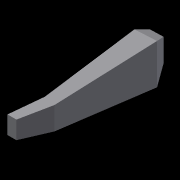
# Autodesk Inventor part: DistalPhalangeIndexMiddle
Saved by Autodesk Inventor 2015 (Build 190159000, 159)
## iProperties
RuleStatus: InUse
Created: 2014-10-29
Part Number: DistalPhalangeIndexMiddle
Material: Generic
Document SubType Name: Modeling
Designer: Val
Density: 1 g/cm^3
Appearance: Default
Mass: 0.761858 g
Surface Area: 6.75236 cm^2
Volume: 0.761858 cm^3
BeforeDocSave0: UpdateBoundingBox
CX: 5.00 mm
CY: 32.00 mm
CZ: 9.00 mm
Author: Val
Autodesk Inventor part; units mm, degrees
ref_plane "YZ Plane" through (0, 0, 0) normal (1, 0, 0) x (0, 1, 0)
ref_plane "XZ Plane" through (0, 0, 0) normal (0, 1, 0) x (-1, 0, 0)
ref_plane "XY Plane" through (0, 0, 0) normal (0, 0, 1) x (1, 0, 0)
sketch "Base" plane through (0, 0, 0) normal (0, 0, 1) x (1, 0, 0)
  line L0 (0, 0) -> (0, -32) construction
  line L1 (0, -32) -> (2, -32)
  line L2 (2, -32) -> (4, -25.4641)
  line L3 (5, -3.4641) -> (3, 0)
  line L4 (3, 0) -> (0, 0)
  line L5 (4, -25.4641) -> (5, -3.4641)
  line L6 (0, -32) -> (1.3607, -25)
  line L7 (1.3607, -25) -> (0, 0)
  dimension "d0" = 32
  dimension "d1" = 3
  dimension "d2" = 2
  dimension "d3" = 5
  dimension "d8" = 4
  dimension "d12" = 120
  dimension "d14" = 22
  dimension "d23" = 25
  dimension "d24" = 79
  constraints: 16 end point, 1 parallel, 1 perpendicular, 1 vertical
  measures "d0" distance of L0.start L0.end
  measures "d1" distance of L3.end L0.start
  measures "d2" distance of L0.end L1.end
  measures "d3" distance from line of L3.start L0
  measures "d8" distance from line of L2.end L0
  measures "d12" angle of L3 L4
  measures "d14" vertical distance of L2.end L3.start
  measures "d23" vertical distance of L6.end L0.start
  measures "d24" angle of L6 L1
extrude "BaseFeature" add sketch "Base" along normal blind 9
sketch "TopProfile" plane through (1.3607, -25, 0) normal (-0.9985, -0.0543, 0) x (0, 0, 1)
  line L0 (0, 21.3063) -> (9, 21.3063) projected
  line L1 (2, 25.037) -> (7, 25.037)
  line L2 (7, 25.037) -> (9, 21.3063)
  line L3 (9, 21.3063) -> (6.5, -7.0244)
  line L4 (6.5, -7.0244) -> (2.5, -7.0244)
  line L5 (2.5, -7.0244) -> (0, 21.3063)
  line L6 (0, 21.3063) -> (2, 25.037)
  line L7 (0, 25.037) -> (9, 25.037) projected
  line L8 (0, -7.0244) -> (9, -7.0244) projected
  point P0 (4.5, 25.037)
  point P1 (4.5, -7.0244)
  dimension "d27" = 5
  dimension "d28" = 4
  constraints: 12 end point, 4 midpoint, 2 collinear, 1 horizontal, 1 parallel
  measures "d27" distance of L1.end L1.start
  measures "d28" distance of L3.end L4.end
extrude "TopProfileFeature" cut sketch "TopProfile" along normal through all both and the other way through all keep common part
